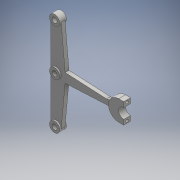
# Autodesk Inventor part: T di connessione
Saved by Autodesk Inventor 2016 (Build 200138000, 138)
## iProperties
Created: 2016-12-03
Part Number: T di connessione
Material: Generic
Document SubType Name: Modeling
Designer: Muhammad
Density: 1 g/cm^3
Appearance: Default
Author: Muhammad
Autodesk Inventor part; units mm, degrees
ref_plane "YZ Plane" through (0, 0, 0) normal (1, 0, 0) x (0, 1, 0)
ref_plane "XZ Plane" through (0, 0, 0) normal (0, 1, 0) x (-1, 0, 0)
ref_plane "XY Plane" through (0, 0, 0) normal (0, 0, 1) x (1, 0, 0)
sketch "Sketch1" plane through (0, 0, 0) normal (0, 1, 0) x (-1, 0, 0)
  circle A0 centre (0, 0) radius 6
  line L0 (0, 0) -> (0, -54.5) construction
  circle A1 centre (0, -54.5) radius 6
  line L1 (0, 0) -> (0, 54.5)
  circle A2 centre (0, 54.5) radius 6
  line L2 (6, 54.5) -> (6, -54.5)
  line L3 (23.6143, 54.5) -> (0, 54.5) construction
  line L4 (0, 54.5) -> (-20.1068, 54.5) construction
  arc A3 (-7.383, 40.137) -> (8.4294, 54.5) centre (-6, 54.5) ccw construction
  line L5 (-6, 54.5) -> (-7.383, 40.137) construction
  line L6 (-6, 54.5) -> (8.4294, 54.5) construction
  line L7 (-6, 54.5) -> (-11.2478, 0)
  line L8 (-6, -54.5) -> (-11.2478, 0)
  arc A4 (-16.1038, 5.1842) -> (16.1245, 6) centre (0, 6) ccw construction
  line L9 (0, 6) -> (-16.1038, 5.1842) construction
  line L10 (0, 6) -> (16.1245, 6) construction
  line L11 (0, 0) -> (-75.5, 0) construction
  line L12 (-10.7223, 5.4568) -> (-63.8233, 2.7668)
  line L13 (-11.2478, 0) -> (-10.7223, -5.4568) construction
  line L14 (-63.5, 0) -> (-63.5, 2.7832) construction
  line L15 (-63.5, 0) -> (-63.5, -2.783) construction
  line L16 (-10.7223, -5.4568) -> (-63.8272, -2.783)
  line L17 (-75.5, 0) -> (-81.5, 0)
  line L18 (-81.5, 0) -> (-81.5, 12)
  line L19 (-81.5, 12) -> (-75.5, 12)
  line L20 (-81.5, 0) -> (-81.5, -12)
  line L21 (-81.5, -12) -> (-75.5, -12)
  arc A5 (-75.5, -12) -> (-75.5, 12) centre (-75.5, 0) ccw
  arc A6 (-87.5, 0) -> (-87.3933, -1.5965) centre (-75.5, 0) ccw
  dimension "d0" = 12
  dimension "d1" = 54.5
  dimension "d2" = 12
  dimension "d5" = 95.5
  dimension "d6" = 177.1
  dimension "d7" = 75.5
  dimension "d9" = 5.482
  dimension "d10" = 2.783
  constraints: 44 end point, 15 point on circle, 14 point on line, 7 centre point, 4 coincident, 4 horizontal, 4 tangent, 2 perpendicular, 2 vertical
  measures "d0" diameter of A0
  measures "d1" distance of L0.start L0.end
  measures "d2" diameter of A1
  measures "d5" angle of L5 L6
  measures "d6" angle of L9 L10
  measures "d7" distance of L0.start L11.end
  measures "d9" distance of L7.end L13.end
  measures "d10" distance of L14.start L15.end
extrude "Extrusion1" add sketch "Sketch1" along normal mid plane 4.5 contours A0 | L2 A1 L8 L7 A2 L1 A0 | A0 L1 A2 L2 | A2 | A1 | L7 L8 L16 A5 L12
sketch "Sketch2" plane through (0, 0, 0) normal (0, 1, 0) x (-1, 0, 0)
  circle A0 centre (0, 0) radius 6
  line L0 (0, 0) -> (0, -54.5) construction
  circle A1 centre (0, -54.5) radius 6
  line L1 (0, 0) -> (0, 54.5)
  circle A2 centre (0, 54.5) radius 6
  line L2 (6, 54.5) -> (6, -54.5)
  line L3 (0, 54.5) -> (-20.1068, 54.5) construction
  arc A3 (-7.383, 40.137) -> (8.4294, 54.5) centre (-6, 54.5) ccw construction
  line L4 (-6, 54.5) -> (-7.383, 40.137) construction
  line L5 (-6, 54.5) -> (8.4294, 54.5) construction
  line L6 (-6, 54.5) -> (-11.2478, 0)
  line L7 (-6, -54.5) -> (-11.2478, 0)
  arc A4 (-16.1038, 5.1842) -> (16.1245, 6) centre (0, 6) ccw construction
  line L8 (0, 6) -> (-16.1038, 5.1842) construction
  line L9 (0, 6) -> (16.1245, 6) construction
  line L10 (0, 0) -> (-75.5, 0) construction
  line L11 (-10.7223, 5.4568) -> (-63.8233, 2.7668)
  line L12 (-11.2478, 0) -> (-10.7223, -5.4568) construction
  line L13 (-63.5, 0) -> (-63.5, 2.7832) construction
  line L14 (-63.5, 0) -> (-63.5, -2.783) construction
  line L15 (-10.7223, -5.4568) -> (-63.8272, -2.783)
  line L16 (-75.5, 0) -> (-81.5, 0)
  line L17 (-81.5, 0) -> (-81.5, 12)
  line L18 (-81.5, 12) -> (-75.5, 12)
  line L19 (-81.5, 0) -> (-81.5, -12)
  line L20 (-81.5, -12) -> (-75.5, -12)
  arc A5 (-75.5, -12) -> (-75.5, 12) centre (-75.5, 0) ccw
  arc A6 (-87.5, 0) -> (-87.3933, -1.5965) centre (-75.5, 0) ccw
  dimension "d14" = 12
  dimension "d15" = 54.5
  dimension "d16" = 12
  dimension "d17" = 95.5
  dimension "d18" = 177.1
  dimension "d19" = 75.5
  dimension "d20" = 5.482
  dimension "d21" = 2.783
  constraints: 42 end point, 15 point on circle, 13 point on line, 7 centre point, 4 coincident, 4 tangent, 3 horizontal, 2 perpendicular, 2 vertical
  measures "d14" diameter of A0
  measures "d15" distance of L1.start L0.end
  measures "d16" diameter of A1
  measures "d17" angle of L4 L5
  measures "d18" angle of L8 L9
  measures "d19" distance of L1.start L10.end
  measures "d20" distance of L6.end L12.end
  measures "d21" distance of L13.start L14.end
extrude "Extrusion2" add sketch "Sketch2" along normal mid plane 8 contours A0 | A2 | A1 | A5 L20 L19 L17 L18
sketch "Sketch3" plane through (0, 4, 0) normal (0, 1, 0) x (1, 0, 0)
  line L0 (81.5, -12) -> (81.5, 12) projected
  circle A0 centre (81.5, 0) radius 6
  point P0 (0, 0)
  dimension "d24" = 12
  constraints: 1 centre point, 1 midpoint
  measures "d24" diameter of A0
extrude "Extrusion3" cut sketch "Sketch3" against normal through all
fillet "Fillet1" radius 6 2 edges at (63.8233, 0, 2.7668) (63.8272, 0, -2.783)
sketch "Sketch4" plane through (0, 4, 54.5) normal (0, 1, 0) x (1, 0, 0)
  circle A0 centre (0, 0) radius 3
  circle A1 centre (0, 54.5) radius 3
  circle A2 centre (0, 109) radius 6 projected
  circle A3 centre (0, 109) radius 3
  dimension "d28" = 6
  dimension "d29" = 6
  dimension "d30" = 6
  constraints: 3 centre point, 2 coincident
  measures "d28" diameter of A0
  measures "d29" diameter of A1
  measures "d30" diameter of A3
extrude "Extrusion4" cut sketch "Sketch4" against normal through all contours A0 | A1 | A3
sketch "Sketch5" plane through (81.5, -4, -12) normal (1, 0, 0) x (0, 0, -1)
  line L0 (-12, 4) -> (-2.5, 4) construction
  circle A0 centre (-2.5, 4) radius 1.5
  line L1 (-12, 11.0799) -> (-12, -3.5917)
  circle A1 centre (-21.5, 4) radius 1.5
  dimension "d33" = 9.5
  constraints: 4 end point, 2 centre point, 1 coincident, 1 horizontal, 1 symmetric about line, 1 vertical, 1 other
  measures "d33" distance of L0.start L0.end
hole "Hole1" at (81.5, 0, 9.5) at (81.5, 0, -9.5) direction (-1, 0, 0) diameter 2.5 depth 10 tip angle 118 counterbore diameter 3 counterbore depth 8
fillet "Fillet2" radius 0.002 29 edges at (8.3612, 2.25, 29.9784) (62.7683, 2.25, 3.7055) (35.1575, 2.25, 4.219) (62.7683, -2.25, 3.7055) (35.1575, -2.25, 4.219) (8.3612, -2.25, 29.9784) (62.7751, 2.25, -3.7192) (35.1626, 2.25, -4.2262) (8.3612, 2.25, -29.9784) (8.3612, -2.25, -29.9784) (6, 4, 0) (78.5, 4, 12) (78.5, 4, -12) (63.5, 4, 0) (75.5, 4, 0) (75.5, -4, 0) (63.5, -4, 0) (78.5, -4, -12) (78.5, -4, 12) (-6, 2.25, 27.25) (-6, 2.25, -27.25) (-6, 4, -54.5) (-6, -4, -54.5) (6, 4, 54.5) (6, -4, 54.5) (81.5, 0, 12) (81.5, 0, 6) (81.5, 0, -6) (81.5, 0, -12)
body "Solid1"
